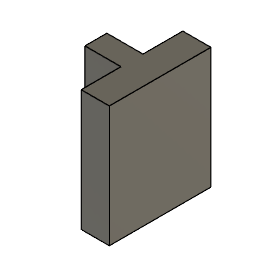
Button Pin (Autodesk Fusion 360 design; units mm, degrees)
Autodesk Fusion 360 part; units mm, degrees
sketch "Sketch5" plane through (0, 0, 0) normal (0, 0, 1) x (1, 0, 0)
  line L0 (1.15, 4.15) -> (-1.15, 4.15)
  line L1 (-1.15, -4.15) -> (1.15, -4.15)
  line L2 (1.15, -4.15) -> (1.15, 4.15)
  line L3 (1.15, 4.15) -> (-1.15, -4.15) construction
  line L4 (-1.15, 4.15) -> (1.15, -4.15) construction
  line L5 (-4.1, 0.9) -> (-4.1, -0.9)
  line L6 (-4.1, -0.9) -> (-1.15, -0.9)
  line L7 (1.15, -0.9) -> (1.15, 0.9)
  line L8 (-1.15, 0.9) -> (-4.1, 0.9)
  line L9 (-1.15, 4.15) -> (-1.15, 0.9)
  line L10 (-1.15, -0.9) -> (-1.15, -4.15)
  dimension "d16" = 2.3
  dimension "d17" = 8.3
  dimension "d18" = 1.8
  dimension "d20" = 2.95
  constraint horizontal L0
  constraint perpendicular L0 L9
  constraint parallel L0 L1
  constraint parallel L2 L9
  constraint coincident L3 origin
  constraint coincident L4 origin
  constraint vertical L5
  constraint horizontal L6
  constraint vertical L7
  constraint coincident L2 L7.end
  constraint collinear L9 L10
  measures "d16" distance of L0.start L0.end
  measures "d17" distance of L0.start L1.end
  measures "d18" distance of L5.start L5.end
  measures "d20" distance of L5.end L6.end
extrude "Extrude4" add sketch "Sketch5" along normal blind 9.892
equation "d16 = 2.5 mm - 0.2 mm"
equation "d17 = 8.60 mm - 0.3 mm"
equation "d18 = 2 mm - 0.2 mm"
equation "d20 = 3.05 mm - 0.1 mm"
equation "d21 = 8.092 mm - 0.2 mm + 2 mm"
